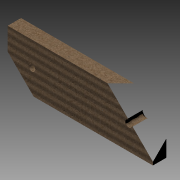
# Autodesk Inventor part: Link
Saved by Autodesk Inventor 2014 SP1 (Build 180222100, 222)
## iProperties
Created: 2014-01-12
Part Number: Link
Material: MDF Medium Density Fiberboard
Document SubType Name: Modeling
Designer: tuleu
Density: 0.8 g/cm^3
Appearance: Cardboard - Corrugated
Author: tuleu
Autodesk Inventor part; units mm, degrees
ref_plane "YZ Plane" through (0, 0, 0) normal (1, 0, 0) x (0, 1, 0)
ref_plane "XZ Plane" through (0, 0, 0) normal (0, 1, 0) x (-1, 0, 0)
ref_plane "XY Plane" through (0, 0, 0) normal (0, 0, 1) x (1, 0, 0)
sketch "Sketch1" plane through (0, 0, 0) normal (0, 1, 0) x (-1, 0, 0)
  line L0 (60, 20) -> (-60, 20)
  line L1 (-60, 20) -> (-60, -20)
  line L2 (-60, -20) -> (60, -20)
  line L3 (60, -20) -> (60, 20)
  line L4 (0, 0) -> (-60, 0) construction
  line L5 (0, 0) -> (0, -20) construction
  dimension "d0" = 120
  dimension "d1" = 40
  constraints: 12 end point, 3 perpendicular, 2 midpoint, 2 parallel, 1 horizontal, 2 other
  measures "d0" distance of L1.end L2.end
  measures "d1" distance of L2.end L0.start
extrude "Extrusion1" add sketch "Sketch1" along normal mid plane 16
sketch "Sketch2" plane through (0, 8, 0) normal (0, 1, 0) x (1, 0, 0)
  line L0 (-60, -20) -> (60, -20) projected
  line L1 (60, -20) -> (60, 20) projected
  line L2 (60, 20) -> (-60, 20) projected
  line L3 (-60, 20) -> (-60, -20) projected
  circle A0 centre (-40, 0) radius 2.75
  circle A1 centre (40, 0) radius 2.75
  line L4 (-60, 0) -> (60, 0) construction
  line L5 (0, 20) -> (0, -20) construction
  point P0 (0, 0)
  dimension "d5" = 5.5
  dimension "d7" = 40
  constraints: 4 end point, 4 midpoint, 2 centre point, 2 point on line, 1 equal radius, 1 symmetric about line
  measures "d5" diameter of A0
  measures "d7" distance of point (0, 0) A0.centre
extrude "Extrusion2" cut sketch "Sketch2" against normal through all contours A0 | A1
chamfer "Chamfer1" distance 5 angle 45 4 edges at (-60, 8, 0) (0, 8, 20) (0, 8, -20) (60, 8, 0)
chamfer "Chamfer2" distance 2 angle 45 2 edges at (-42.75, 8, 0) (37.25, 8, 0)
body "Solid1"
